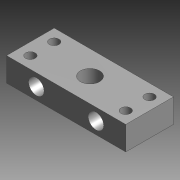
# Autodesk Inventor part: montura tensor
Saved by Autodesk Inventor 2011 (Build 150239000, 239)
## iProperties
Created: 2010-04-23
Part Number: montura tensor
Document SubType Name: Modeling
Designer: lucio
Density: 1 g/cm^3
Author: lucio
Autodesk Inventor part; units mm, degrees
ref_plane "YZ Plane" through (0, 0, 0) normal (1, 0, 0) x (0, 1, 0)
ref_plane "XZ Plane" through (0, 0, 0) normal (0, 1, 0) x (-1, 0, 0)
ref_plane "XY Plane" through (0, 0, 0) normal (0, 0, 1) x (1, 0, 0)
sketch "Sketch1" plane through (0, 0, 0) normal (0, 0, 1) x (1, 0, 0)
  line L0 (-18.9222, 4.1916) -> (31.0778, 4.1916)
  line L1 (31.0778, 4.1916) -> (31.0778, -15.8084)
  line L2 (31.0778, -15.8084) -> (-18.9222, -15.8084)
  line L3 (-18.9222, -15.8084) -> (-18.9222, 4.1916)
  dimension "d2" = 50
  dimension "d3" = 20
  constraints: 8 end point, 2 parallel, 1 horizontal, 1 perpendicular
  measures "d2" distance of L1.end L2.end
  measures "d3" distance of L0.end L1.end
extrude "Extrusion1" add sketch "Sketch1" along normal blind 10
sketch "Sketch2" plane through (-18.9222, -15.8084, 0) normal (0, -1, 0) x (1, 0, 0)
  line L0 (0, 0) -> (0, 10) projected
  line L1 (50, 0) -> (50, 10) projected
  point P0 (18.9222, 0)
  point P1 (12.5, 5)
  point P2 (37.5, 5)
  dimension "d6" = 12.5
  dimension "d7" = 12.5
  dimension "d35" = 50
  measures "d6" distance from line of L0 point (12.5, 5)
  measures "d7" distance from line of L1 point (37.5, 5)
  measures "d35" distance of L1.start L0.start
hole "Hole1" at (-6.4222, -15.8084, 5) at (18.5778, -15.8084, 5) direction (0, 1, 0) diameter 6.5 end through all
sketch "Sketch3" plane through (0, 0, 10) normal (0, 0, 1) x (1, 0, 0)
  line L0 (31.0778, 4.1916) -> (31.0778, -15.8084) projected
  line L1 (31.0778, -15.8084) -> (-18.9222, -15.8084) projected
  point P0 (0, 0)
  point P1 (6.0778, -5.8084)
  dimension "d36" = 20
  dimension "d37" = 50
  dimension "d38" = 25
  dimension "d39" = 10
  measures "d36" distance of L0.start L0.end
  measures "d37" distance of L0.end L1.end
  measures "d38" distance from line of L0 point (6.078, -5.808)
  measures "d39" distance from line of L1 point (6.078, -5.808)
hole "Hole2" at (6.0778, -5.8084, 10) direction (0, 0, -1) diameter 8 end through all
sketch "Sketch4" plane through (0, 0, 10) normal (0, 0, 1) x (1, 0, 0)
  line L0 (-18.9222, -15.8084) -> (-18.9222, 4.1916) projected
  line L1 (31.0778, -15.8084) -> (-18.9222, -15.8084) projected
  line L2 (-13.9222, -0.8084) -> (26.0778, -0.8084)
  line L3 (26.0778, -0.8084) -> (26.0778, -10.8084)
  line L4 (26.0778, -10.8084) -> (-13.9222, -10.8084)
  line L5 (-13.9222, -10.8084) -> (-13.9222, -0.8084)
  point P0 (31.0778, 4.1916)
  point P1 (0, 0)
  dimension "d22" = 50
  dimension "d23" = 40
  dimension "d24" = 10
  dimension "d25" = 20
  dimension "d26" = 5
  dimension "d27" = 5
  constraints: 8 end point, 2 parallel, 1 horizontal, 1 perpendicular
  measures "d22" distance of L0.end point (31.078, 4.192)
  measures "d23" distance of L2.start L2.end
  measures "d24" distance of L4.end L2.start
  measures "d25" distance of L0.start L0.end
  measures "d26" distance between parallel lines of L1 L4
  measures "d27" distance between parallel lines of L0 L5
hole "Hole3" at (-13.9222, -0.8084, 10) at (26.0778, -0.8084, 10) at (26.0778, -10.8084, 10) at (-13.9222, -10.8084, 10) direction (0, 0, -1) diameter 4 end through all
equation "\"d6\" = d7"
equation "\"d7\" = 0.25 * d35"
equation "\"d38\" = 0.5 * d37"
equation "\"d39\" = 0.5 * d36"
equation "\"d26\" = -0.5 * d24 + 0.5 * d25"
equation "\"d27\" = -0.5 * d23 + 0.5 * d22"
body "Solid1"
